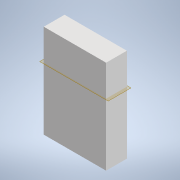
# Autodesk Inventor part: esp32CAM
Saved by Autodesk Inventor 2020 (Build 240168000, 168)
## iProperties
Created: 2022-12-14
Part Number: esp32CAM
Material: Generic
Document SubType Name: Modeling
Designer: Manish
Density: 1 g/cm^3
Appearance: Default
Author: Manish
Autodesk Inventor part; units mm, degrees
ref_plane "YZ Plane" through (0, 0, 0) normal (1, 0, 0) x (0, 1, 0)
ref_plane "XZ Plane" through (0, 0, 0) normal (0, 1, 0) x (-1, 0, 0)
ref_plane "XY Plane" through (0, 0, 0) normal (0, 0, 1) x (1, 0, 0)
sketch "Sketch1" plane through (0, 0, 0) normal (0, 0, 1) x (1, 0, 0)
  line L0 (0, 0) -> (0, -45)
  line L1 (0, -45) -> (30, -45)
  line L2 (30, -45) -> (30, 0)
  line L3 (30, 0) -> (0, 0)
  dimension "d0" = 45
  dimension "d1" = 30
  constraints: 8 end point, 2 parallel, 1 perpendicular, 1 vertical
  measures "d0" distance of L0.start L0.end
  measures "d1" distance of L1.end L0.end
extrude "Extrusion1" add sketch "Sketch1" against normal blind 10
sketch "Sketch2" plane through (0, 0, -10) normal (0, 0, -1) x (-1, 0, 0)
  line L0 (0, 0) -> (-30, 0) projected
  line L1 (-15, 0) -> (-15, -45)
  line L2 (-30, -45) -> (0, -45) projected
  line L3 (0, -45) -> (0, 0) projected
  line L4 (0, -22.5) -> (-30, -22.5)
  line L5 (-30, 0) -> (-30, -45) projected
  circle A0 centre (-15, -15) radius 5
  dimension "d4" = 10
  dimension "d5" = 15
  constraints: 4 end point, 4 midpoint, 1 centre point, 1 point on line
  measures "d4" diameter of A0
  measures "d5" distance from line of A0.centre L0
extrude "Extrusion2" add sketch "Sketch2" along normal blind 5 contours A0 L1 | L1 A0
ref_plane "Work Plane1" through (0, -15, 0) normal (0, 1, 0) x (1, 0, 0)
body "Solid1"
